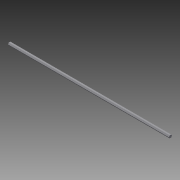
# Autodesk Inventor part: back roller 7-16 hex shaft
Saved by Autodesk Inventor 2015 SP1 (Build 190203100, 203)
## iProperties
Created: 2015-01-15
Part Number: back roller 7-16 hex shaft
Material: Generic
Document SubType Name: Modeling
Designer: 215152
Density: 1 g/cm^3
Appearance: Default
Author: 215152
Autodesk Inventor part; units mm, degrees
ref_plane "YZ Plane" through (0, 0, 0) normal (1, 0, 0) x (0, 1, 0)
ref_plane "XZ Plane" through (0, 0, 0) normal (0, 1, 0) x (-1, 0, 0)
ref_plane "XY Plane" through (0, 0, 0) normal (0, 0, 1) x (1, 0, 0)
sketch "Sketch1" plane through (0, 0, 0) normal (1, 0, 0) x (0, 1, 0)
  line L0 (5.5563, 3.2079) -> (5.5563, -3.2079)
  line L1 (5.5563, -3.2079) -> (0, -6.4158)
  line L2 (0, -6.4158) -> (-5.5563, -3.2079)
  line L3 (-5.5563, -3.2079) -> (-5.5563, 3.2079)
  line L4 (-5.5563, 3.2079) -> (0, 6.4158)
  line L5 (0, 6.4158) -> (5.5563, 3.2079)
  point P0 (0, 0)
  dimension "d0" = 11.1125
  dimension "d1" = 11.1125
  dimension "d2" = 11.1125
  dimension "d3" = 5.5563
  dimension "d4" = 120
  dimension "d5" = 120
  dimension "d6" = 5.5563
  dimension "d7" = 5.5563
  constraints: 12 end point, 3 parallel, 1 vertical
  measures "d0" distance between parallel lines of L3 L0
  measures "d1" distance between parallel lines of L4 L1
  measures "d2" distance between parallel lines of L2 L5
  measures "d3" distance from line of point (0, 0) L0
  measures "d4" angle of L0 L5
  measures "d5" angle of L1 L0
  measures "d6" distance from line of point (0, 0) L1
  measures "d7" distance from line of point (0, 0) L5
extrude "Extrusion1" add sketch "Sketch1" along normal blind 685.8
body "Solid1"
